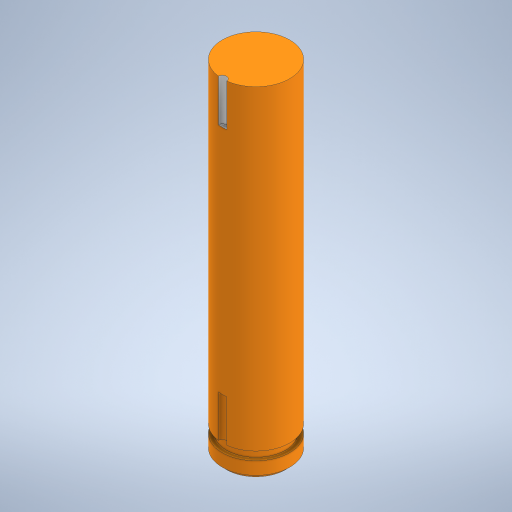
# Autodesk Inventor part: Trục
Saved by Autodesk Inventor 2023 (Build 270158000, 158)
## iProperties
Created: 2023-10-05
Part Number: Trục
Material: Generic
Document SubType Name: Modeling
Designer: huy20
Density: 1 g/cm^3
Appearance: Default
Author: huy20
Autodesk Inventor part; units mm, degrees
ref_plane "YZ Plane" through (0, 0, 0) normal (1, 0, 0) x (0, 1, 0)
ref_plane "XZ Plane" through (0, 0, 0) normal (0, 1, 0) x (-1, 0, 0)
ref_plane "XY Plane" through (0, 0, 0) normal (0, 0, 1) x (1, 0, 0)
sketch "Sketch1" plane through (0, 0, 0) normal (0, 1, 0) x (-1, 0, 0)
  circle A0 centre (0, 0) radius 4
  dimension "d0" = 8
  constraints: 1 centre point, 1 coincident
  measures "d0" diameter of A0
extrude "Extrusion1" add sketch "Sketch1" along normal blind 40.5
chamfer "Chamfer1" distance 0.5 angle 45 1 edges at (4, 0, 0)
sketch "Sketch2" plane through (0, 0, 0) normal (0, 0, 1) x (1, 0, 0)
  line L0 (-4, 0.5) -> (-4, 40.5) construction
  line L1 (-3.5, 0) -> (-4, 0.5) construction
  line L2 (-4, 0.5) -> (4, 0.5) construction
  line L3 (3.5, 0) -> (-3.5, 0) construction
  line L4 (4, 40.5) -> (-4, 40.5) projected
  line L5 (-4, 0.5) -> (4, 0.5) construction
  line L6 (3.5, 0) -> (4, 0.5) construction
  line L7 (4, 0.5) -> (4, 40.5) construction
  line L8 (4, 3) -> (3.5, 3)
  line L9 (3.5, 3) -> (3.5, 2)
  line L10 (3.5, 2) -> (4, 2)
  line L11 (4, 2) -> (4, 3)
  line L12 (0, -7.9) -> (0, 47.4) projected
  point P0 (0, 0)
  dimension "d6" = 2
  dimension "d7" = 1
  dimension "d8" = 0.5
  constraints: 8 end point, 2 parallel, 1 horizontal, 1 perpendicular, 1 point on line
  measures "d6" distance between parallel lines of L10 L3
  measures "d7" distance between parallel lines of L8 L10
  measures "d8" distance between parallel lines of L7 L9
revolve "Revolution1" cut sketch "Sketch2" angle 360 about axis through (0, -10, 0) along (0, 1, 0)
sketch "Sketch6" plane through (0, 3, 0) normal (0, -1, 0) x (1, 0, 0)
  circle A0 centre (0, 0) radius 3.5 construction
  circle A1 centre (0, 0) radius 4 construction
  circle A2 centre (0, 0) radius 4 projected
  circle A3 centre (0, 4) radius 0.5
  constraints: 1 centre point, 1 tangent, 1 vertical alignment, 1 other
extrude "Extrusion4" cut sketch "Sketch6" against normal blind 5 contours A3 A2 | A2 A3 picked at (0.0193, 3.8321) picked at (0.0153, 4.1636)
sketch "Sketch7" plane through (0, 40.5, 0) normal (0, 1, 0) x (1, 0, 0)
  arc A0 (0.499, -3.9688) -> (-0.499, -3.9688) centre (0, -4) ccw projected
  circle A1 centre (0, -4) radius 0.5
  point P0 (0, 0)
  point P1 (-0.499, -3.9688)
  point P2 (0.499, -3.9688)
  constraints: 1 centre point, 1 coincident
extrude "Extrusion5" cut sketch "Sketch7" against normal blind 5
body "Solid1"
